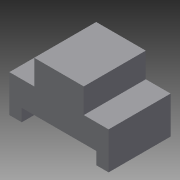
# Autodesk Inventor part: 7.1 Part 2
Saved by Autodesk Inventor 2015 (Build 190159000, 159)
## iProperties
Created: 2015-03-05
Part Number: 7.1 Part 2
Material: Generic
Document SubType Name: Modeling
Designer: PLTW-Stu-02
Density: 1 g/cm^3
Appearance: Default
Author: PLTW-Stu-02
Autodesk Inventor part; units mm, degrees
ref_plane "YZ Plane" through (0, 0, 0) normal (1, 0, 0) x (0, 1, 0)
ref_plane "XZ Plane" through (0, 0, 0) normal (0, 1, 0) x (-1, 0, 0)
ref_plane "XY Plane" through (0, 0, 0) normal (0, 0, 1) x (1, 0, 0)
sketch "Sketch1" plane through (0, 0, 0) normal (0, 0, 1) x (1, 0, 0)
  line L0 (68.7422, 12.7568) -> (68.7422, 31.8068)
  line L1 (56.0422, 44.5068) -> (30.6422, 44.5068)
  line L2 (17.9422, 31.8068) -> (17.9422, 12.7568)
  line L3 (17.9422, 31.8068) -> (30.6422, 31.8068)
  line L4 (30.6422, 31.8068) -> (30.6422, 44.5068)
  line L5 (68.7422, 31.8068) -> (56.0422, 31.8068)
  line L6 (56.0422, 31.8068) -> (56.0422, 44.5068)
  line L7 (24.2922, 12.7568) -> (24.2922, 19.1068)
  line L8 (24.2922, 19.1068) -> (62.3922, 19.1068)
  line L9 (62.3922, 19.1068) -> (62.3922, 12.7568)
  line L10 (17.9422, 12.7568) -> (24.2922, 12.7568)
  line L11 (62.3922, 12.7568) -> (68.7422, 12.7568)
  point P0 (0, 0)
  constraints: 24 end point, 7 perpendicular, 4 horizontal, 3 parallel, 1 vertical
extrude "Extrusion1" add sketch "Sketch1" along normal blind 31.75
body "Solid1"
